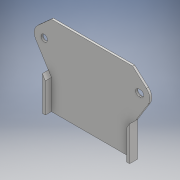
# Autodesk Inventor part: mini5電腦支架
Saved by Autodesk Inventor 2017 (Build 210142000, 142)
## iProperties
Part Number: mini5電腦支架
Material: 一般
Document SubType Name: Modeling
Designer: user
Density: 1 g/cm^3
Appearance: 預設
Author: user
Autodesk Inventor part; units mm, degrees
ref_plane "YZ Plane" through (0, 0, 0) normal (1, 0, 0) x (0, 1, 0)
ref_plane "XZ Plane" through (0, 0, 0) normal (0, 1, 0) x (-1, 0, 0)
sketch "草圖1" plane through (0, 0, 0) normal (0, 1, 0) x (-1, 0, 0)
  line L0 (0, 0) -> (-80.6, 0)
  line L1 (-80.6, 0) -> (-80.6, 79.4)
  line L2 (-80.6, 79.4) -> (0, 79.4)
  line L3 (0, 79.4) -> (0, 0)
  line L4 (-80.6, 79.4) -> (-80.6, 51.023)
  line L5 (-80.6, 79.4) -> (-80.6, 51.023)
  line L6 (-80.6, 51.023) -> (-80.6, 79.4)
  line L7 (-94.3269, 67.1422) -> (-80.6, 79.4)
  line L8 (-96.1567, 54.4) -> (-80.6, 29.4)
  circle A0 centre (-87.6663, 59.6833) radius 3.25
  arc A1 (-94.3269, 67.1422) -> (-96.1567, 54.4) centre (-87.6663, 59.6833) ccw
  line L9 (-40.2, 92.1708) -> (-40.2, -8.9293) construction
  line L10 (0, 79.4) -> (13.727, 67.142)
  line L11 (15.5567, 54.3998) -> (0, 29.3998)
  circle A2 centre (7.0663, 59.6831) radius 3.25
  arc A3 (15.5567, 54.3998) -> (13.727, 67.142) centre (7.0663, 59.6831) ccw
  point P0 (-100.6, 61.5405)
  point P1 (20, 61.5403)
  point P2 (17.5946, 57.6964)
  point P3 (10.5946, 57.6964)
  dimension "d0" = 80.6
  dimension "d1" = 79.4
  dimension "d7" = 50
  dimension "d10" = 20
  dimension "d11" = 6.5
  dimension "d12" = 10
  dimension "d13" = 25
  dimension "d17" = 20
  dimension "d18" = 6.5
  dimension "d19" = 10
  dimension "d20" = 25
  dimension "d42" = 7
  dimension "d51" = 13.727
  constraints: 24 end point, 7 point on line, 4 centre point, 4 point on circle, 4 tangent, 2 coincident, 2 collinear, 2 parallel, 1 horizontal, 1 perpendicular, 1 vertical
  measures "d0" distance of L1.end L2.end
  measures "d1" distance of L0.end L1.end
  measures "d7" distance of L8.end L1.end
  measures "d10" distance from line of point (-100.6, 61.541) L4
  measures "d11" diameter of A0
  measures "d12" radius of A1
  measures "d13" vertical distance of L8.start L8.end
  measures "d17" distance from line of L3 point (20, 61.54)
  measures "d18" diameter of A2
  measures "d19" radius of A3
  measures "d20" vertical distance of L11.start L11.end
  measures "d42" distance of point (17.595, 57.696) point (10.595, 57.696)
  measures "d51" horizontal distance of L2.end L10.end
extrude "擠出1" add sketch "草圖1" along normal blind 2
sketch "草圖11" plane through (0, 2, 0) normal (0, 1, 0) x (1, 0, 0)
  circle A0 centre (87.6663, -59.6833) radius 3.25 construction
  line L0 (88.4163, -62.9333) -> (86.9163, -62.9333)
  line L1 (83.6663, -59.6833) -> (83.6663, -59.6833)
  line L2 (86.9163, -56.4333) -> (88.4163, -56.4333)
  line L3 (91.6663, -59.6833) -> (91.6663, -59.6833)
  arc A1 (88.4163, -62.9333) -> (91.6663, -59.6833) centre (88.4163, -59.6833) ccw
  arc A2 (91.6663, -59.6833) -> (88.4163, -56.4333) centre (88.4163, -59.6833) ccw
  arc A3 (86.9163, -56.4333) -> (83.6663, -59.6833) centre (86.9163, -59.6833) ccw
  arc A4 (83.6663, -59.6833) -> (86.9163, -62.9333) centre (86.9163, -59.6833) ccw
  point P0 (0, 0)
  dimension "d46" = 4
  dimension "d47" = 4
  dimension "d48" = 3.25
  constraints: 10 tangent, 8 end point, 8 point on circle, 4 centre point, 3 equal radius, 2 parallel, 1 horizontal, 1 perpendicular
  measures "d46" distance from line of A0.centre L3
  measures "d47" distance from line of L1 A0.centre
  measures "d48" radius of A1
extrude "擠出5" cut sketch "草圖11" against normal through all
sketch "草圖18" plane through (0, 2, 0) normal (0, 1, 0) x (1, 0, 0)
  line L0 (0, 0) -> (-3, 0)
  line L1 (0, -29.3998) -> (-15.5567, -54.3998) projected
  line L2 (0, 0) -> (0, -29.3998) projected
  line L3 (-3, 0) -> (-3, -34.2209)
  line L4 (40.2999, -89.2199) -> (40.2999, 11.3236) construction
  line L5 (80.5999, 0) -> (83.5999, 0)
  line L6 (80.5999, 0) -> (80.5999, -29.3998)
  line L7 (83.5999, 0) -> (83.5999, -34.2209)
  line L8 (96.1567, -54.4) -> (80.6, -29.4) projected
  line L9 (83.5999, -34.2209) -> (80.6, -29.4)
  dimension "d60" = 3
  constraints: 14 end point, 4 symmetric about line, 2 vertical, 1 collinear, 1 horizontal, 1 point on line
  measures "d60" distance of L0.start L0.end
extrude "擠出7" add sketch "草圖18" against normal blind 8 contours L2 L1 L3 L0
ref_plane "工作平面4" through (40.3, -6, 29.3998) normal (1, 0, 0) x (0, 0, -1)
mirror "鏡射2" about plane through (40.3, -6, 29.3998) normal (1, 0, 0) of "擠出7"
